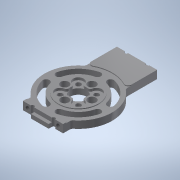
# Autodesk Inventor part: 付け根ロール_メインフレーム_1_1
Saved by Autodesk Inventor 2020.4 (Build 244396000, 396)
## iProperties
Created: 2016-05-01
Part Number: 付け根ロール_メインフレーム_1_1
Material: アルミニウム 2014-T4
Document SubType Name: Modeling
Designer: hiroaki
Density: 2.8 g/cm^3
Appearance: 滑らか - 淡い灰色
Mass: 20.3148 g
Surface Area: 78.5669 cm^2
Volume: 7.25528 cm^3
Category: 付け根
Author: hiroaki
Autodesk Inventor part; units mm, degrees
ref_plane "YZ Plane" through (0, 0, 0) normal (1, 0, 0) x (0, 1, 0)
ref_plane "XZ Plane" through (0, 0, 0) normal (0, 1, 0) x (-1, 0, 0)
ref_plane "XY Plane" through (0, 0, 0) normal (0, 0, 1) x (1, 0, 0)
derived "付け根ロール_基礎.ipt"
sketch "スケッチ1" plane through (0, 0, 0) normal (0, 0, 1) x (1, 0, 0)
  circle A0 centre (0, 0) radius 5.05 projected
  circle A1 centre (0, -8.5) radius 1.35 projected
  circle A2 centre (0, -8.5) radius 2.5 projected
  circle A3 centre (-5.6569, -5.6569) radius 1.55 projected
  line L0 (-5.6569, -5.6569) -> (0, 0) construction
  line L1 (0, 0) -> (0, -8.5) construction
  line L2 (-4.835, -8.7241) -> (-7.9022, -7.9022) construction
  line L3 (-7.9022, -7.9022) -> (-8.7241, -4.835) construction
  line L4 (-8.7241, -4.835) -> (-6.4787, -2.5896) construction
  line L5 (-6.4787, -2.5896) -> (-3.4115, -3.4115) construction
  line L6 (-3.4115, -3.4115) -> (-2.5896, -6.4787) construction
  line L7 (-2.5896, -6.4787) -> (-4.835, -8.7241) construction
  circle A4 centre (5.6569, -5.6569) radius 1.55 projected
  line L8 (8.7241, -4.835) -> (7.9022, -7.9022) construction
  line L9 (7.9022, -7.9022) -> (4.835, -8.7241) construction
  line L10 (4.835, -8.7241) -> (2.5896, -6.4787) construction
  line L11 (3.4115, -3.4115) -> (6.4787, -2.5896) construction
  line L12 (2.5896, -6.4787) -> (3.4115, -3.4115) construction
  line L13 (6.4787, -2.5896) -> (8.7241, -4.835) construction
  circle A5 centre (8.5, 0) radius 2.5 projected
  circle A6 centre (8.5, 0) radius 1.35 projected
  circle A7 centre (5.6569, 5.6569) radius 1.55 projected
  line L14 (4.835, 8.7241) -> (7.9022, 7.9022) construction
  line L15 (7.9022, 7.9022) -> (8.7241, 4.835) construction
  line L16 (8.7241, 4.835) -> (6.4787, 2.5896) construction
  line L17 (3.4115, 3.4115) -> (2.5896, 6.4787) construction
  line L18 (6.4787, 2.5896) -> (3.4115, 3.4115) construction
  line L19 (2.5896, 6.4787) -> (4.835, 8.7241) construction
  circle A8 centre (0, 8.5) radius 2.5 projected
  circle A9 centre (0, 8.5) radius 1.35 projected
  circle A10 centre (-5.6569, 5.6569) radius 1.55 projected
  line L20 (-8.7241, 4.835) -> (-7.9022, 7.9022) construction
  line L21 (-7.9022, 7.9022) -> (-4.835, 8.7241) construction
  line L22 (-4.835, 8.7241) -> (-2.5896, 6.4787) construction
  line L23 (-3.4115, 3.4115) -> (-6.4787, 2.5896) construction
  line L24 (-2.5896, 6.4787) -> (-3.4115, 3.4115) construction
  line L25 (-6.4787, 2.5896) -> (-8.7241, 4.835) construction
  circle A11 centre (-8.5, 0) radius 2.5 projected
  circle A12 centre (-8.5, 0) radius 1.35 projected
  circle A13 centre (0, 0) radius 12.45 construction
  circle A14 centre (0, 0) radius 21 construction
  line L26 (-12.5, 36.5) -> (-12.5, -22) construction
  line L27 (-12.5, -22) -> (-7.6, -22)
  line L28 (-12.5, 36.5) -> (-7.6, 36.5)
  line L29 (7.6, 36.5) -> (12.5, 36.5)
  line L30 (12.5, 36.5) -> (12.5, -22) construction
  line L31 (12.5, -22) -> (7.6, -22)
  line L32 (0, 0) -> (0, 8.5) construction
  line L33 (-5.5, 36.5) -> (-5.5, 38.5)
  line L34 (-5.5, 38.5) -> (5.5, 38.5)
  line L35 (5.5, 38.5) -> (5.5, 36.5)
  line L36 (-5.5, -22) -> (-5.5, -24)
  line L37 (-5.5, -24) -> (5.5, -24)
  line L38 (5.5, -24) -> (5.5, -22)
  arc A15 (-7.6, 36.5) -> (-5.5, 36.5) centre (-6.55, 36.5) ccw
  line L39 (-7.6, 36.5) -> (-5.5, 36.5) construction
  line L40 (-5.5, 36.5) -> (-5.5, 36.5) construction
  arc A16 (5.5, 36.5) -> (7.6, 36.5) centre (6.55, 36.5) ccw
  arc A17 (-5.5, -22) -> (-7.6, -22) centre (-6.55, -22) ccw
  arc A18 (7.6, -22) -> (5.5, -22) centre (6.55, -22) ccw
  line L41 (-11.05, 38.5) -> (-7.95, 38.5) construction
  line L42 (-7.95, 38.5) -> (-7.95, 35.1002) construction
  line L43 (-7.95, 35.1002) -> (-11.05, 35.1002) construction
  line L44 (-11.05, 35.1002) -> (-11.05, 38.5) construction
  line L45 (-9.5, 38.5) -> (-9.5, 35.1002) construction
  line L46 (12.5, 7.25) -> (-12.5, 7.25) construction
  line L47 (-12.5, -22) -> (-12.5, -16.8745)
  arc A19 (-12.5, 16.8745) -> (-12.5, -16.8745) centre (0, 0) ccw
  line L48 (-12.5, 16.8745) -> (-12.5, 36.5)
  line L49 (12.5, -22) -> (12.5, -16.8745)
  arc A20 (12.5, -16.8745) -> (12.5, 16.8745) centre (0, 0) ccw
  line L50 (12.5, 36.5) -> (12.5, 16.8745)
  circle A21 centre (0, 24.25) radius 3.25 construction
  circle A22 centre (0, 24.25) radius 1.05 projected
  circle A23 centre (-24.25, 0) radius 1.05 projected
  circle A24 centre (0, -24.25) radius 1.05 projected
  circle A25 centre (24.25, 0) radius 1.05 projected
  line L51 (2.75, 25.8377) -> (2.75, 22.6623) projected
  line L52 (2.75, 22.6623) -> (0, 21.0746) projected
  line L53 (0, 21.0746) -> (-2.75, 22.6623) projected
  line L54 (-2.75, 22.6623) -> (-2.75, 25.8377) projected
  line L55 (-2.75, 25.8377) -> (0, 27.4254) projected
  line L56 (0, 27.4254) -> (2.75, 25.8377) projected
  dimension "d22" = 1.05
  dimension "d23" = 25
  dimension "d24" = 58.5
  dimension "d25" = 2
  dimension "d26" = 2
  dimension "d27" = 22
  dimension "d28" = 7
  dimension "d29" = 3.1
  dimension "d30" = 3
  constraints: 50 end point, 15 point on circle, 9 perpendicular, 6 centre point, 6 symmetric about line, 5 collinear, 5 midpoint, 4 horizontal, 4 tangent, 4 vertical, 3 parallel, 2 coincident, 1 equal radius, 1 vertical alignment, 4 other
  measures "d22" radius of A15
  measures "d23" distance between parallel lines of L26 L30
  measures "d24" distance of L29.end L30.end
  measures "d25" distance between parallel lines of L29 L34
  measures "d26" distance between parallel lines of L37 L31
  measures "d27" distance from line of A14.centre L31
  measures "d28" distance between parallel lines of L33 L26
  measures "d29" distance of L41.start L41.end
  measures "d30" distance between parallel lines of L26 L45
extrude "押し出し1" add sketch "スケッチ1" along normal blind 5 contours L47 A19 L48 L28 A15 L33 L34 L35 A16 L29 L50 A20 L49 L31 A18 L38 L37 A24 L36 A17 L27 | A24 L37 | A22 | L51 L52 L53 L54 L55 L56 picked at (0.0124, -23.6569)
sketch "スケッチ3" plane through (-12.5, -22, 0) normal (0, -1, 0) x (1, 0, 0)
  line L0 (0, 0) -> (0, 5) projected
  line L1 (12.5, 0) -> (12.5, 8.5841) construction
  point P0 (3, 2.5)
  point P1 (22, 2.5)
  point P2 (0, 2.5)
  dimension "d33" = 3
  constraints: 2 end point, 1 horizontal alignment, 1 midpoint, 1 symmetric about line, 1 vertical
  measures "d33" distance from line of L0 point (3, 2.5)
hole "穴1" at (-9.5, -22, 2.5) at (9.5, -22, 2.5) direction (0, 1, 0) diameter 2.459 depth 2.5 thread size "M3x0.5" class "6H" standard "ISO Metric profile"
sketch "スケッチ4" plane through (7.6, 36.5, 0) normal (0, 1, 0) x (1, 0, 0)
  line L0 (4.9, 0) -> (4.9, -5) projected
  line L1 (-7.6, 0) -> (-7.6, -11.9426) construction
  point P0 (-17.1, -2.5)
  point P1 (1.9, -2.5)
  point P2 (4.9, -2.5)
  dimension "d41" = 3
  constraints: 2 end point, 1 horizontal alignment, 1 midpoint, 1 symmetric about line, 1 vertical
  measures "d41" distance from line of L0 point (1.9, -2.5)
hole "穴2" at (-9.5, 36.5, 2.5) at (9.5, 36.5, 2.5) direction (0, -1, 0) diameter 2.459 depth 2.5 thread size "M3x0.5" class "6H" standard "ISO Metric profile"
sketch "スケッチ6" plane through (-5.5, -24, 5) normal (0, 0, 1) x (1, 0, 0)
  line L0 (-2.1, 60.5) -> (-7, 60.5) projected
  line L1 (-7, 2) -> (-2.1, 2) projected
  line L2 (-3.4142, -3.7238) -> (17.6304, -3.7238)
  line L3 (17.6304, -3.7238) -> (17.6304, 2)
  line L4 (17.6304, 2) -> (-3.4142, 2)
  line L5 (-3.4142, 2) -> (-3.4142, -3.7238)
  line L6 (-1.5604, 60.5) -> (14.161, 60.5)
  line L7 (14.161, 60.5) -> (14.161, 68.3853)
  line L8 (14.161, 68.3853) -> (-1.5604, 68.3853)
  line L9 (-1.5604, 68.3853) -> (-1.5604, 60.5)
  constraints: 16 end point, 4 parallel, 2 collinear, 2 horizontal, 2 perpendicular
extrude "押し出し3" cut sketch "スケッチ6" against normal blind 2.5
sketch "スケッチ7" plane through (7.6, -22, 5) normal (0, 0, 1) x (1, 0, 0)
  arc A0 (4.9, 5.1255) -> (4.9, 38.8745) centre (-7.6, 22) ccw projected
  circle A1 centre (-13.2569, 16.3431) radius 1.55 construction
  circle A2 centre (-13.2569, 27.6569) radius 1.55 projected
  circle A3 centre (-1.9431, 27.6569) radius 1.55 projected
  circle A4 centre (-1.9431, 16.3431) radius 1.55 projected
  line L0 (-14.0937, 19.4661) -> (-10.9707, 18.6293) construction
  line L1 (-10.9707, 18.6293) -> (-10.1339, 15.5063) construction
  line L2 (-10.1339, 15.5063) -> (-12.4201, 13.2202) construction
  line L3 (-12.4201, 13.2202) -> (-15.543, 14.057) construction
  line L4 (-15.543, 14.057) -> (-16.3798, 17.1799) construction
  line L5 (-16.3798, 17.1799) -> (-14.0937, 19.4661) construction
  line L6 (-12.4201, 13.2202) -> (-15.543, 14.057) construction
  line L7 (-15.543, 14.057) -> (-16.3798, 17.1799) construction
  line L8 (-16.3798, 17.1799) -> (-14.0937, 19.4661) construction
  line L9 (-14.0937, 19.4661) -> (-10.9707, 18.6293) construction
  line L10 (-10.9707, 18.6293) -> (-10.1339, 15.5063) construction
  line L11 (-10.1339, 15.5063) -> (-12.4201, 13.2202) construction
  line L12 (-13.2569, 16.3431) -> (-10.9707, 18.6293) construction
  circle A5 centre (-7.6, 22) radius 5.05 projected
  line L13 (-10.9707, 18.6293) -> (-7.6, 22) construction
  circle A6 centre (-13.2569, 16.3431) radius 3.2332
  circle A7 centre (-1.9431, 16.3431) radius 3.2332
  circle A8 centre (-1.9431, 27.6569) radius 3.2332
  circle A9 centre (-13.2569, 27.6569) radius 3.2332
  point P0 (-15.493, 14.057)
  point P1 (-12.3701, 13.2202)
  point P2 (-10.0839, 15.5063)
  point P3 (-10.9207, 18.6293)
  point P4 (-14.0437, 19.4661)
  point P5 (1.1798, 17.1799)
  point P6 (-2.7799, 30.7798)
  point P7 (-16.3798, 26.8201)
  dimension "d67" = 5.6
  dimension "d99" = 5.6
  dimension "d102" = 360
  constraints: 28 end point, 6 collinear, 2 coincident, 38 other
  measures "d67" distance between parallel lines of L3 L0
  measures "d99" distance between parallel lines of L6 L9
extrude "押し出し4" cut sketch "スケッチ7" against normal blind 1.5 contours A4 | A8 A5 | A5 A8 | A7 A5 | A5 A7 | A9 A5 | A5 A9 | A6 A5 | A5 A6
sketch "スケッチ8" plane through (7.6, -22, 5) normal (0, 0, 1) x (1, 0, 0)
  arc A0 (4.9, 5.1255) -> (4.9, 38.8745) centre (-7.6, 22) ccw projected
  circle A1 centre (-7.6, 22) radius 5.05 projected
  circle A2 centre (-7.6, 22) radius 12.45
  circle A3 centre (-7.6, 22) radius 21.05
  dimension "d79" = 24.9
  dimension "d82" = 0.05
  constraints: 2 centre point, 2 coincident
  measures "d79" diameter of A2
  measures "d82" radial gap between concentric circles of A3 A0
extrude "押し出し5" cut sketch "スケッチ8" against normal blind 0.5 contours A3
sketch "スケッチ10" plane through (7.6, -22, 4.5) normal (0, 0, 1) x (1, 0, 0)
  arc A0 (4.9, 5.1255) -> (4.9, 38.8745) centre (-7.6, 22) ccw projected
  arc A1 (-20.1, 38.8745) -> (-20.1, 5.1255) centre (-7.6, 22) ccw projected
  circle A2 centre (-7.6, 22) radius 12.45 projected
  arc A3 (-25.9916, 20) -> (-9.6, 3.6084) centre (-7.6, 22) ccw
  line L0 (-25.9916, 20) -> (-21.9109, 20)
  line L1 (-9.6, 3.6084) -> (-9.6, 7.6891)
  arc A4 (-21.9109, 20) -> (-9.6, 7.6891) centre (-7.6, 22) ccw
  arc A5 (-5.6, 3.6084) -> (10.7916, 20) centre (-7.6, 22) ccw
  line L2 (-5.6, 3.6084) -> (-5.6, 7.6891)
  line L3 (10.7916, 20) -> (6.7109, 20)
  arc A6 (-5.6, 7.6891) -> (6.7109, 20) centre (-7.6, 22) ccw
  arc A7 (10.7916, 24) -> (-5.6, 40.3916) centre (-7.6, 22) ccw
  line L4 (10.7916, 24) -> (6.7109, 24)
  line L5 (-5.6, 40.3916) -> (-5.6, 36.3109)
  arc A8 (6.7109, 24) -> (-5.6, 36.3109) centre (-7.6, 22) ccw
  arc A9 (-9.6, 40.3916) -> (-25.9916, 24) centre (-7.6, 22) ccw
  line L6 (-9.6, 40.3916) -> (-9.6, 36.3109)
  line L7 (-25.9916, 24) -> (-21.9109, 24)
  arc A10 (-9.6, 36.3109) -> (-21.9109, 24) centre (-7.6, 22) ccw
  dimension "d88" = 2.5
  dimension "d89" = 2
  dimension "d90" = 2
  dimension "d91" = 2
  dimension "d94" = 360
  constraints: 16 end point, 16 point on circle, 8 centre point, 2 coincident, 1 horizontal, 1 vertical, 41 other
  measures "d88" radial gap between concentric circles of A1 A3
  measures "d89" radial gap between concentric circles of A4 A2
  measures "d90" distance from line of A0.centre L0
  measures "d91" distance from line of A0.centre L1
extrude "押し出し7" cut sketch "スケッチ10" against normal blind 5 contours L0 A4 L1 A3 | L2 A6 L3 A5 | L4 A8 L5 A7 | L6 A10 L7 A9
fillet "フィレット2" radius 2 20 edges at (-12.5, -16.9367, 4.75) (12.5, -16.9367, 4.75) (2, -18.3916, 2.25) (2, -14.3109, 2.25) (-2, -18.3916, 2.25) (-2, -14.3109, 2.25) (14.3109, -2, 2.25) (18.3916, -2, 2.25) (18.3916, 2, 2.25) (14.3109, 2, 2.25) (2, 14.3109, 2.25) (2, 18.3916, 2.25) (-2, 18.3916, 2.25) (-2, 14.3109, 2.25) (-18.3916, -2, 2.25) (-14.3109, -2, 2.25) (-18.3916, 2, 2.25) (-14.3109, 2, 2.25) (12.5, 16.9367, 4.75) (-12.5, 16.9367, 4.75)
fillet "フィレット3" radius 1.5 8 edges at (-4.2328, 2.7542, 4.25) (-4.2328, -2.7542, 4.25) (2.7542, 4.2328, 4.25) (4.2328, 2.7542, 4.25) (4.2328, -2.7542, 4.25) (2.7542, -4.2328, 4.25) (-2.7542, -4.2328, 4.25) (-2.7542, 4.2328, 4.25)
fillet "フィレット4" radius 2.1 4 edges at (12.5, -16.8745, 2.25) (12.5, 16.8745, 2.25) (-12.5, 16.8745, 2.25) (-12.5, -16.8745, 2.25)
equation "\"d26\" = d25"
equation "\"d28\" = d17 + d18"
equation "\"d30\" = d17"
equation "\"d33\" = d17"
equation "\"d41\" = d17"
equation "\"d91\" = d90"
equation "\"d17\" = 3"
equation "\"d18\" = 4"
